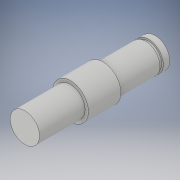
# Autodesk Inventor part: Stage1_carrier_shaft
Saved by Autodesk Inventor 2019 (Build 230136000, 136)
## iProperties
Created: 2019-12-31
Part Number: Stage1_carrier_shaft
Material: 一般
Document SubType Name: Modeling
Designer: user
Density: 1 g/cm^3
Appearance: 預設
Author: user
Autodesk Inventor part; units mm, degrees
ref_plane "YZ Plane" through (0, 0, 0) normal (1, 0, 0) x (0, 1, 0)
ref_plane "XZ Plane" through (0, 0, 0) normal (0, 1, 0) x (-1, 0, 0)
ref_plane "XY Plane" through (0, 0, 0) normal (0, 0, 1) x (1, 0, 0)
sketch "草圖2" plane through (0, 0, 0) normal (0, 0, 1) x (1, 0, 0)
  circle A0 centre (0, 0) radius 4.5
  dimension "d3" = 9
  constraints: 1 centre point, 1 coincident
  measures "d3" diameter of A0
extrude "擠出2" add sketch "草圖2" along normal blind 40
ref_plane "工作平面3" through (0, 0, 16) normal (0, 0, -1) x (-1, 0, 0)
sketch "草圖5" plane through (0, 0, 16) normal (0, 0, -1) x (-1, 0, 0)
  circle A0 centre (0, 0) radius 5.5
  dimension "d15" = 11
  constraints: 1 centre point, 1 coincident
  measures "d15" diameter of A0
extrude "擠出5" add sketch "草圖5" against normal blind 10
ref_plane "工作平面4" through (0, 0, 2) normal (0, 0, -1) x (-1, 0, 0)
sketch "草圖6" plane through (0, 0, 2) normal (0, 0, -1) x (-1, 0, 0)
  circle A0 centre (0, 0) radius 4
  circle A1 centre (0, 0) radius 4.5 projected
  dimension "d19" = 8
  constraints: 1 centre point, 1 coincident
  measures "d19" diameter of A0
extrude "擠出6" cut sketch "草圖6" against normal blind 1
